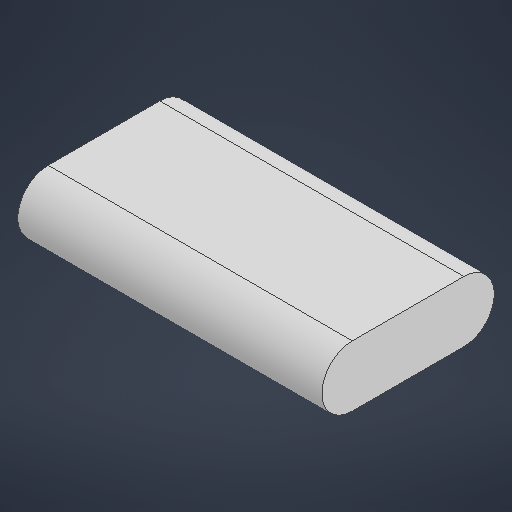
# Autodesk Inventor part: Battery_prop
Saved by Autodesk Inventor 2027 (Build 310192060, 192F)
## iProperties
Created: 2026-06-27
Part Number: Battery_prop
Material: Ogólny
Document SubType Name: Modeling
Designer: User
Density: 1 g/cm^3
Appearance: Domyślna
Author: User
Autodesk Inventor part; units mm, degrees
ref_plane "YZ Plane" through (0, 0, 0) normal (1, 0, 0) x (0, 1, 0)
ref_plane "XZ Plane" through (0, 0, 0) normal (0, 1, 0) x (-1, 0, 0)
ref_plane "XY Plane" through (0, 0, 0) normal (0, 0, 1) x (1, 0, 0)
sketch "Szkic1" plane through (0, 0, 0) normal (0, 1, 0) x (-1, 0, 0)
  line L0 (-15, -8.5) -> (15, -8.5)
  line L1 (15, -8.5) -> (15, 8.5)
  line L2 (15, 8.5) -> (-15, 8.5)
  line L3 (-15, 8.5) -> (-15, -8.5)
  line L4 (-15, -8.5) -> (15, 8.5) construction
  line L5 (15, -8.5) -> (-15, 8.5) construction
  point P0 (0, 0)
  dimension "d0" = 30
  dimension "d1" = 17
  constraints: 12 end point, 2 midpoint, 2 parallel, 1 horizontal, 1 perpendicular
  measures "d0" distance of L2.end L1.end
  measures "d1" distance of L1.end L0.end
extrude "Wyciągnięcie proste1" add sketch "Szkic1" along normal blind 6
fillet "Zaokrąglenie1" radius 3 4 edges at (0, 6, 8.5) (0, 0, 8.5) (0, 6, -8.5) (0, 0, -8.5)
